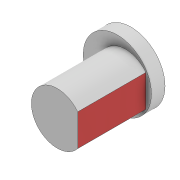
# Autodesk Inventor part: input
Saved by Autodesk Inventor 2022 (Build 260153000, 153)
## iProperties
Created: 2023-11-18
Part Number: input
Material: 一般
Document SubType Name: Modeling
Designer: JOU
Density: 1 g/cm^3
Appearance: 預設
Author: JOU
Autodesk Inventor part; units mm, degrees
ref_plane "YZ Plane" through (0, 0, 0) normal (1, 0, 0) x (0, 1, 0)
ref_plane "XZ Plane" through (0, 0, 0) normal (0, 1, 0) x (-1, 0, 0)
ref_plane "XY Plane" through (0, 0, 0) normal (0, 0, 1) x (1, 0, 0)
sketch "草圖1" plane through (0, 0, 0) normal (0, 0, 1) x (1, 0, 0)
  circle A0 centre (0, 0) radius 25
  dimension "d0" = 50
  constraints: 1 centre point, 1 coincident
  measures "d0" diameter of A0
extrude "擠出1" add sketch "草圖1" along normal blind 10
sketch "草圖2" plane through (0, 0, 10) normal (0, 0, 1) x (1, 0, 0)
  circle A0 centre (6, 0) radius 19
  circle A1 centre (0, 0) radius 25 projected
  dimension "d3" = 6
  constraints: 1 centre point, 1 horizontal alignment, 1 tangent
  measures "d3" distance of point (0, 0) A0.centre
extrude "擠出2" add sketch "草圖2" along normal blind 50 contours A0
sketch "草圖3" plane through (6, 0, 60) normal (0, 0, 1) x (1, 0, 0)
  circle A0 centre (0, 0) radius 19 projected
  circle A1 centre (0, 0) radius 19 projected
  line L0 (15, 11.6619) -> (15, -11.6619)
  point P0 (-6, 0)
  point P1 (19, 0)
  point P2 (15, 11.6619)
  point P3 (15, -11.6619)
  dimension "d6" = 15
  constraints: 2 end point, 2 point on circle, 1 vertical, 1 other
  measures "d6" distance from line of L0 point (0, 0)
extrude "擠出3" cut sketch "草圖3" against normal up to surface (50 mm away) contours A0 L0 picked at (16.3333, 0)
